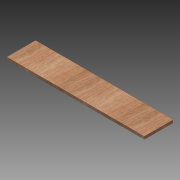
# Autodesk Inventor part: sectional_wasteboard
Saved by Autodesk Inventor 2013 SP2 (Build 170200200, 200)
## iProperties
Created: 2013-05-31
Part Number: sectional_wasteboard
Material: Wood (Birch)
Document SubType Name: Modeling
Designer: Edward
Density: 0.55 g/cm^3
Description: 12.7mm x 600mm x 125mm MDF blanks
Vendor: custom
Mass: 523.875 g
Surface Area: 1684.15 cm^2
Volume: 952.5 cm^3
Stock Number: SM_WB
Author: Edward
Autodesk Inventor part; units mm, degrees
ref_plane "YZ Plane" through (0, 0, 0) normal (1, 0, 0) x (0, 1, 0)
ref_plane "XZ Plane" through (0, 0, 0) normal (0, 1, 0) x (-1, 0, 0)
ref_plane "XY Plane" through (0, 0, 0) normal (0, 0, 1) x (1, 0, 0)
sketch "Sketch1" plane through (0, 0, 0) normal (0, 0, 1) x (1, 0, 0)
  line L0 (-300, -62.5) -> (300, -62.5)
  line L1 (300, -62.5) -> (300, 62.5)
  line L2 (300, 62.5) -> (-300, 62.5)
  line L3 (-300, 62.5) -> (-300, -62.5)
  point P0 (0, 0)
  dimension "d0" = 600
  dimension "d1" = 125
  dimension "d2" = 300
  dimension "d3" = 62.5
  constraints: 8 end point, 2 parallel, 1 horizontal, 1 perpendicular
  measures "d0" distance of L2.end L1.end
  measures "d1" distance of L1.end L0.end
  measures "d2" distance from line of L3 point (0, 0)
  measures "d3" distance from line of L2 point (0, 0)
extrude "Extrusion1" add sketch "Sketch1" along normal blind 12.7
equation "\"d2\" = 0.5 * d0"
equation "\"d3\" = 0.5 * d1"
body "Solid1"
